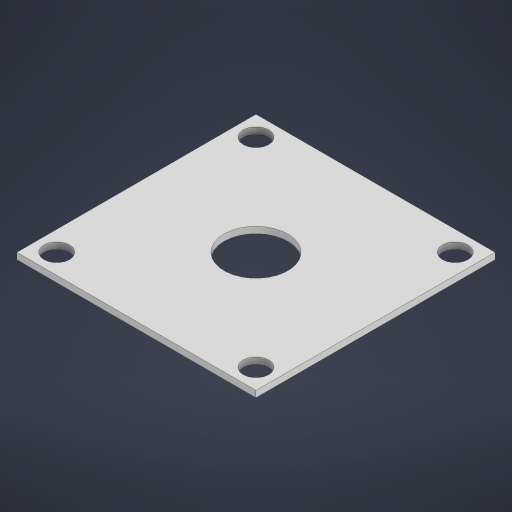
# Autodesk Inventor part: Base
Saved by Autodesk Inventor 2023 (Build 270158000, 158)
## iProperties
Created: 2023-03-04
Part Number: Base
Material: 一般
Document SubType Name: Modeling
Designer: neko2
Density: 1 g/cm^3
Appearance: 既定
Author: neko2
Autodesk Inventor part; units mm, degrees
ref_plane "YZ Plane" through (0, 0, 0) normal (1, 0, 0) x (0, 1, 0)
ref_plane "XZ Plane" through (0, 0, 0) normal (0, 1, 0) x (-1, 0, 0)
ref_plane "XY Plane" through (0, 0, 0) normal (0, 0, 1) x (1, 0, 0)
sketch "スケッチ1" plane through (0, 0, 0) normal (0, 1, 0) x (-1, 0, 0)
  line L0 (-15, -15) -> (15, -15)
  line L1 (15, -15) -> (15, 15)
  line L2 (15, 15) -> (-15, 15)
  line L3 (-15, 15) -> (-15, -15)
  line L4 (-15, -15) -> (15, 15) construction
  line L5 (15, -15) -> (-15, 15) construction
  circle A0 centre (0, 0) radius 4
  dimension "d0" = 30
  dimension "d1" = 30
  dimension "d2" = 8
  constraints: 12 end point, 2 midpoint, 2 parallel, 1 centre point, 1 coincident, 1 horizontal, 1 perpendicular
  measures "d0" distance of L2.end L1.end
  measures "d1" distance of L1.end L0.end
  measures "d2" diameter of A0
extrude "押し出し1" add sketch "スケッチ1" along normal blind 0.8
sketch "スケッチ2" plane through (0, 0.8, 0) normal (0, 1, 0) x (1, 0, 0)
  circle A0 centre (-12.5, -12.5) radius 1.6
  line L0 (0, -18.82) -> (0, 21.247)
  line L1 (-16.0432, 0) -> (16.9483, 0)
  circle A1 centre (-12.5, 12.5) radius 1.6
  circle A2 centre (12.5, -12.5) radius 1.6
  circle A3 centre (12.5, 12.5) radius 1.6
  line L2 (-15, 15) -> (-15, -15) projected
  line L3 (-15, -15) -> (15, -15) projected
  point P0 (0, 0)
  dimension "d5" = 3.2
  dimension "d10" = 25
  dimension "d13" = 25
  dimension "d18" = 2.5
  dimension "d19" = 2.5
  constraints: 4 centre point, 4 end point, 2 horizontal, 2 point on line, 2 vertical, 6 other
  measures "d5" diameter of A0
  measures "d10" distance of A0.centre A1.centre
  measures "d13" distance of A0.centre A2.centre
  measures "d18" distance from line of A0.centre L2
  measures "d19" distance from line of L3 A0.centre
extrude "押し出し2" cut sketch "スケッチ2" against normal through all contours A0 | A1 | A2 | A3
